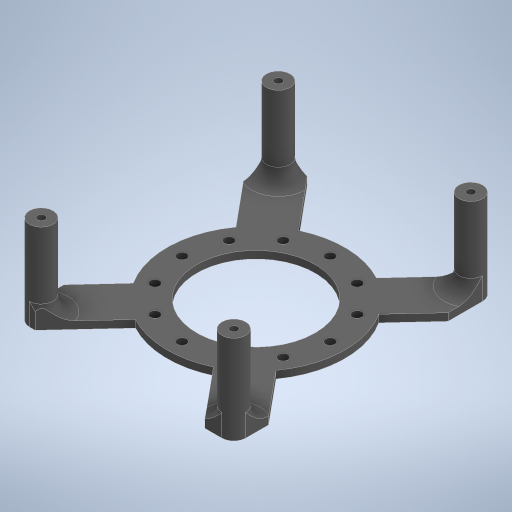
# Autodesk Inventor part: board_base_connect
Saved by Autodesk Inventor 2024.1 (Build 281209000, 209)
## iProperties
Created: 2024-08-02
Part Number: board_base_connect
Material: 一般
Document SubType Name: Modeling
Designer: hibik
Density: 1 g/cm^3
Appearance: 既定
Author: hibik
Autodesk Inventor part; units mm, degrees
ref_plane "YZ Plane" through (0, 0, 0) normal (1, 0, 0) x (0, 1, 0)
ref_plane "XZ Plane" through (0, 0, 0) normal (0, 1, 0) x (-1, 0, 0)
ref_plane "XY Plane" through (0, 0, 0) normal (0, 0, 1) x (1, 0, 0)
sketch "スケッチ1" plane through (0, 0, 0) normal (0, 1, 0) x (-1, 0, 0)
  line L0 (-32.5, -40) -> (32.5, -40) construction
  line L1 (32.5, -40) -> (32.5, 40) construction
  line L2 (32.5, 40) -> (-32.5, 40) construction
  line L3 (-32.5, 40) -> (-32.5, -40) construction
  line L4 (-32.5, -40) -> (32.5, 40) construction
  line L5 (32.5, -40) -> (-32.5, 40) construction
  circle A0 centre (32.5, 40) radius 4
  circle A1 centre (32.5, -40) radius 4
  circle A2 centre (-32.5, -40) radius 4
  circle A3 centre (-32.5, 40) radius 4
  circle A4 centre (32.5, 40) radius 1.3
  circle A5 centre (32.5, -40) radius 1.3
  circle A6 centre (-32.5, 40) radius 1.3
  circle A7 centre (-32.5, -40) radius 1.3
  point P0 (0, 0)
  dimension "d0" = 65
  dimension "d1" = 80
  dimension "d2" = 8
  dimension "d4" = 2.6
  constraints: 12 end point, 8 centre point, 8 coincident, 6 equal radius, 2 midpoint, 2 parallel, 1 horizontal, 1 perpendicular
  measures "d0" distance of L2.end L1.end
  measures "d1" distance of L1.end L0.end
  measures "d2" diameter of A0
  measures "d4" diameter of A4
extrude "押し出し1" add sketch "スケッチ1" along normal blind 30
sketch "スケッチ2" plane through (32.5, 0, 40) normal (0, -1, 0) x (1, 0, 0)
  circle A0 centre (-32.5, -40) radius 20
  circle A1 centre (-32.5, -40) radius 30
  circle A2 centre (-32.5, -15) radius 1.6
  line L0 (-32.5, -40) -> (-32.5, -10) construction
  line L1 (-32.5, -20) -> (-32.5, -10)
  circle A3 centre (-45, -18.3494) radius 1.6
  circle A4 centre (-54.1506, -27.5) radius 1.6
  circle A5 centre (-57.5, -40) radius 1.6
  circle A6 centre (-54.1506, -52.5) radius 1.6
  circle A7 centre (-45, -61.6506) radius 1.6
  circle A8 centre (-32.5, -65) radius 1.6
  circle A9 centre (-20, -61.6506) radius 1.6
  circle A10 centre (-10.8494, -52.5) radius 1.6
  circle A11 centre (-7.5, -40) radius 1.6
  circle A12 centre (-10.8494, -27.5) radius 1.6
  circle A13 centre (-20, -18.3494) radius 1.6
  line L2 (-69, 4) -> (4, 4)
  line L3 (4, 4) -> (4, -84)
  line L4 (4, -84) -> (-69, -84)
  line L5 (-69, -84) -> (-69, 4)
  circle A14 centre (0, 0) radius 4 projected
  circle A15 centre (0, -80) radius 4 projected
  circle A16 centre (-65, -80) radius 4 projected
  circle A17 centre (-65, 0) radius 4 projected
  line L6 (9.7724, -0.7885) -> (-63.2276, -88.7885)
  line L7 (-63.2276, -88.7885) -> (-74.7724, -79.2115)
  line L8 (-74.7724, -79.2115) -> (-1.7724, 8.7885)
  line L9 (-1.7724, 8.7885) -> (9.7724, -0.7885)
  line L10 (9.7724, -0.7885) -> (-74.7724, -79.2115) construction
  line L11 (-63.2276, -88.7885) -> (-1.7724, 8.7885) construction
  line L12 (-76.8175, -3.2514) -> (0.8202, -86.9495)
  line L13 (0.8202, -86.9495) -> (11.8175, -76.7486)
  line L14 (11.8175, -76.7486) -> (-65.8202, 6.9495)
  line L15 (-65.8202, 6.9495) -> (-76.8175, -3.2514)
  line L16 (-76.8175, -3.2514) -> (11.8175, -76.7486) construction
  line L17 (0.8202, -86.9495) -> (-65.8202, 6.9495) construction
  point P0 (-69, 0)
  point P1 (-69, -80)
  point P2 (-65, -84)
  point P3 (0, -84)
  point P4 (4, -80)
  point P5 (4, 0)
  point P6 (0, 4)
  point P7 (-65, 4)
  point P8 (-19.7267, -12.8551)
  point P9 (-46.7555, -13.6034)
  point P10 (-63.0842, 4)
  point P11 (-69, -11.6791)
  point P12 (-57.7527, -23.8044)
  point P13 (-56.8181, -57.5679)
  point P14 (-69, -72.253)
  point P15 (-59.2554, -84)
  point P16 (-45.2733, -67.1449)
  point P17 (-18.2445, -66.3966)
  point P18 (-1.9158, -84)
  point P19 (4, -68.3209)
  point P20 (-7.2473, -56.1956)
  point P21 (-8.1819, -22.4321)
  point P22 (4, -7.747)
  point P23 (-5.7446, 4)
  dimension "d7" = 40
  dimension "d8" = 60
  dimension "d9" = 3.2
  dimension "d12" = 360
  dimension "d17" = 15
  constraints: 36 end point, 12 centre point, 6 midpoint, 6 parallel, 4 perpendicular, 4 tangent, 3 point on line, 2 coincident, 1 collinear, 1 equal length, 1 horizontal, 1 vertical, 1 vertical alignment, 30 other
  measures "d9" diameter of A2
  measures "d17" distance between parallel lines of L8 L6
extrude "押し出し2" add sketch "スケッチ2" against normal blind 2.5 contours A0 L6 A12 A1 L14 A10 | A0 L8 A1 L6 A12 | L14 A10 A1 L12 A0 | A0 L1 A2 A1 L8 | L12 A1 L6 A0 | A0 L14 A1 L1 A2 | L8 L2 A14 L3 L6 A1 | L6 A1 L8 A6 A0 | A1 L14 L3 A15 L4 L12 | A0 L12 A4 A1 L14 | L8 A6 A1 L12 A4 A0 | L6 L4 A16 L5 L8 A1 | A1 L12 L5 A17 L2 L14
fillet "フィレット1" radius 5 6 edges at (-29.6716, 2.5, -37.1716) (-29.6716, 2.5, 37.1716) (32.5, 2.5, 36) (29.6716, 2.5, 42.8284) (29.6716, 2.5, -42.8284) (32.5, 2.5, -36)
